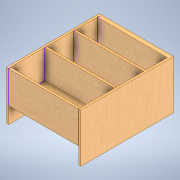
# Autodesk Inventor part: container unit
Saved by Autodesk Inventor 2022.2 (Build 262287000, 287)
## iProperties
Created: 2022-02-26
Part Number: container unit
Material: Pine, Southern
Document SubType Name: Modeling
Designer: PRASHANTH
Density: 0.570257 g/cm^3
Appearance: Yellow Pine - Stained Dark Medium Gloss
Author: PRASHANTH
Autodesk Inventor part; units mm, degrees
ref_plane "YZ Plane" through (0, 0, 0) normal (1, 0, 0) x (0, 1, 0)
ref_plane "XZ Plane" through (0, 0, 0) normal (0, 1, 0) x (-1, 0, 0)
ref_plane "XY Plane" through (0, 0, 0) normal (0, 0, 1) x (1, 0, 0)
sketch "Sketch1" plane through (0, 0, 0) normal (1, 0, 0) x (0, 1, 0)
  line L0 (-22.6931, 110) -> (55.0359, 110)
  line L1 (55, -110) -> (-22.6931, -110)
  line L2 (-62.7298, 0) -> (-22.6931, -110)
  line L3 (-62.7298, 0) -> (-22.6931, 110)
  line L4 (-57.4089, 0) -> (-19.449, -104.2938)
  line L5 (-14.4482, -105) -> (55, -105)
  line L6 (55.0359, 105) -> (-14.4122, 105)
  line L7 (-19.449, 104.2938) -> (-57.4089, 0)
  line L8 (55.0034, 17.6855) -> (-14.4593, 17.6855)
  line L9 (55.0034, 22.5) -> (-14.4456, 22.5496)
  line L10 (55, -52.5) -> (-14.449, -52.5)
  line L11 (55, -47.6855) -> (-14.449, -47.7352)
  line L12 (-60.6224, -5.7899) -> (-60, -7.5)
  line L13 (-60.6224, 5.7899) -> (-60, 7.5)
  line L14 (-14.4122, 105) -> (-14.4122, 68.1255)
  line L15 (-14.4456, 59.4672) -> (-14.4456, 22.5496)
  line L16 (-19.449, 104.2938) -> (-19.449, 68.1255)
  line L17 (-14.4593, 17.6855) -> (-14.4593, -10.5317)
  line L18 (-14.449, -19.4683) -> (-14.449, -47.7352)
  line L19 (-19.4705, 59.4672) -> (-19.4705, -10.5317)
  line L20 (-14.449, -52.5) -> (-14.449, -74.4672)
  line L21 (-14.4482, -83.1255) -> (-14.4482, -105.0928)
  line L22 (-19.4499, -19.4683) -> (-19.4499, -74.4672)
  line L23 (-19.449, -83.1255) -> (-19.449, -104.2938)
  line L24 (-19.449, -74.4672) -> (-19.4499, -74.4672)
  line L25 (-14.4593, -83.1255) -> (-14.4482, -83.1255)
  line L26 (-19.4499, -19.4683) -> (-19.449, -19.4683)
  line L27 (-19.4705, -10.5317) -> (-19.449, -10.5317)
  line L28 (-14.4122, 68.1255) -> (-14.4125, 68.1255)
  line L29 (-19.4705, 59.4672) -> (-19.449, 59.4672)
  line L30 (55.0359, 105) -> (55.0359, 110)
  line L31 (55.0034, 22.5) -> (55.0034, 17.6855)
  line L32 (55, -47.6855) -> (55, -52.5)
  line L33 (55, -105) -> (55, -110)
  line L34 (-19.449, -91.3967) -> (-19.449, 76.5553)
  line L35 (-14.4122, 69.213) -> (-14.4225, 22.5496)
  line L36 (-14.4236, 17.6855) -> (-14.438, -47.7351)
  line L37 (-14.439, -52.5) -> (-14.4482, -94.1091)
  point P0 (0, 0)
  constraints: 76 end point, 32 parallel, 20 point on line, 6 perpendicular, 2 horizontal, 1 midpoint
extrude "Extrusion1" add sketch "Sketch1" along normal blind 170
sketch "Sketch2" plane through (0, -14.4236, 17.6855) normal (0, 1, -0.0002) x (1, 0, 0)
  circle A0 centre (80, 33.4744) radius 10
  circle A1 centre (80, 98.5003) radius 10
  circle A2 centre (80, -44.9284) radius 10
  point P0 (0, 17.6824)
  dimension "d24" = 20
  dimension "d25" = 20
  dimension "d26" = 20
  constraints: 3 centre point
  measures "d24" diameter of A0
  measures "d25" diameter of A1
  measures "d26" diameter of A2
extrude "Extrusion2" cut sketch "Sketch2" against normal blind 6
sketch "Sketch3" plane through (0, -22.6931, -110) normal (0, -0.9397, -0.342) x (1, 0, 0)
  point P0 (0, 95.6047)
sketch "Sketch4" plane through (0, -22.6931, -110) normal (0, -0.9397, -0.342) x (1, 0, 0)
  line L0 (0, 117.1568) -> (170, 117.1568) projected
  circle A0 centre (85, 117.1568) radius 7.5
  point P0 (0, 95.6047)
  dimension "d29" = 15
  constraints: 1 centre point, 1 midpoint
  measures "d29" diameter of A0
extrude "Extrusion3" cut sketch "Sketch4" against normal blind 10
sketch "Sketch5" plane through (0, 0, 0) normal (-1, 0, 0) x (0, 0, 1)
  line L0 (-110, -22.6931) -> (-110, 55) projected
  line L1 (-110, 55) -> (109.7253, 55)
  line L2 (109.7253, 55) -> (109.7253, -62.9244)
  line L3 (109.7253, -62.9244) -> (-110, -62.9244)
  line L4 (-110, -62.9244) -> (-110, 55)
  point P0 (0, 0)
  constraints: 8 end point, 2 parallel, 1 horizontal, 1 perpendicular
extrude "Extrusion4" add sketch "Sketch5" along normal blind 5
sketch "Sketch6" plane through (170, 0, 0) normal (1, 0, 0) x (0, 0, -1)
  line L0 (-109.7253, 55) -> (-109.7253, -22.793) projected
  line L1 (110, -22.6931) -> (110, -62.9244) projected
  line L2 (-109.7253, 55) -> (110, 55)
  line L3 (110, 55) -> (110, -62.9244)
  line L4 (110, -62.9244) -> (-109.7253, -62.9244)
  line L5 (-109.7253, -62.9244) -> (-109.7253, 55)
  point P0 (0, 0)
  constraints: 8 end point, 2 parallel, 1 horizontal, 1 perpendicular
extrude "Extrusion5" add sketch "Sketch6" along normal blind 5
sketch "Sketch7" plane through (0, -62.9244, 109.7253) normal (0, 0, 1) x (1, 0, 0)
  line L0 (-5, 117.9244) -> (175, 117.9244) projected
  line L1 (-5, 117.9244) -> (175, 117.9244)
  line L2 (175, 117.9244) -> (175, 0)
  line L3 (175, 0) -> (-5, 0)
  line L4 (-5, 0) -> (-5, 117.9244)
  line L5 (175, 0) -> (-5, 0)
  line L6 (-5, 0) -> (-5, 117.9244)
  line L7 (-5, 117.9244) -> (175, 117.9244)
  line L8 (175, 117.9244) -> (175, 0)
  point P0 (0, 62.9244)
  constraints: 16 end point, 4 parallel, 2 horizontal, 2 perpendicular
sketch "Sketch8" plane through (0, -22.6931, 110) normal (0, -0.9397, 0.342) x (1, 0, 0)
  circle A0 centre (144.5406, -21.5508) radius 6.0469
  point P0 (0, -95.6047)
  constraints: 1 centre point
extrude "Extrusion6" cut sketch "Sketch8" against normal blind 6
sketch "Sketch9" plane through (0, -62.9244, -110) normal (0, 0, -1) x (-1, 0, 0)
  line L0 (-175, 117.9244) -> (-175, 0) projected
  line L1 (0, 117.9244) -> (5, 117.9244) projected
  line L2 (-175, 0) -> (5, 0)
  line L3 (5, 0) -> (5, 117.9244)
  line L4 (5, 117.9244) -> (-175, 117.9244)
  line L5 (-175, 117.9244) -> (-175, 0)
  point P0 (0, 62.9244)
  point P1 (-175, 117.9244)
  constraints: 8 end point, 2 parallel, 1 horizontal, 1 perpendicular
extrude "Extrusion7" add sketch "Sketch9" along normal blind 5
body "Solid1"
